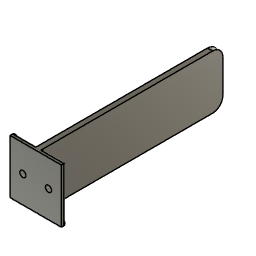
ear_bracket v2 (Autodesk Fusion 360 design; units mm, degrees)
Autodesk Fusion 360 part; units mm, degrees
sketch "Sketch1" plane through (0, 0, 0) normal (0, 1, 0) x (1, 0, 0)
  line L0 (10, -15) -> (-10, -15)
  line L1 (-10, -15) -> (-10, 6)
  line L2 (-10, 6) -> (10, 6)
  line L3 (10, 6) -> (10, -15)
  dimension "d1" = 21
  dimension "d2" = 20
  constraint horizontal L0
  constraint vertical L1
  constraint horizontal L2
  constraint vertical L3
  measures "d1" distance of L0.start L2.end
  measures "d2" distance of L0.start L0.end
extrude "Extrude1" add sketch "Sketch1" along normal blind 2
sketch "Sketch2" plane through (0, 2, 0) normal (0, 1, 0) x (-1, 0, 0)
  line L0 (-10, -6) -> (10, -6)
  line L1 (10, -6) -> (10, 15)
  line L2 (10, 15) -> (-10, 15)
  line L3 (-10, 15) -> (-10, -6)
  line L4 (-1, 15) -> (1, 15)
  line L5 (1, 15) -> (1, -6)
  line L6 (1, -6) -> (-1, -6)
  line L7 (-1, -6) -> (-1, 15)
  dimension "d5" = 2
  dimension "d6" = 9
  constraint horizontal L4
  constraint vertical L5
  constraint horizontal L6
  constraint vertical L7
  constraint coincident L0 L5.end
  constraint coincident L2 L4.start
  measures "d5" distance of L4.start L4.end
  measures "d6" distance of L1 L5
extrude "Extrude2" add sketch "Sketch2" along normal blind 70 contours L0 L2 L4 L5 L6 L7
sketch "Sketch3" plane through (0, 2, 0) normal (0, 1, 0) x (-1, 0, 0)
  line L0 (-1, -6) -> (-1, 15)
  line L1 (-1, 15) -> (-10, 15)
  line L2 (-10, 15) -> (-10, -6)
  line L3 (-10, -6) -> (-1, -6)
  circle A0 centre (-5, 4.5) radius 1.2
  circle A1 centre (5, 4.5) radius 1.2
  line L4 (10, 15) -> (1, 15)
  dimension "d9" = 2.4
  dimension "d10" = 2.4
  dimension "d11" = 10.5
  dimension "d12" = 10.5
  dimension "d19" = 10
  measures "d9" diameter of A0
  measures "d10" diameter of A1
  measures "d11" distance of A1.centre L4
  measures "d12" distance of L1 A0.centre
  measures "d19" distance of A0.centre A1.centre
extrude "Extrude3" cut sketch "Sketch3" against normal blind 2 contours A0 | A1
fillet "Fillet1" radius 1 6 edges at (10, 2, 4.5) (5.5, 2, 15) (-5.5, 2, 15) (-10, 2, 4.5) (-5.5, 2, -6) (5.5, 2, -6)
fillet "Fillet2" radius 4 2 edges at (0, 72, 15) (0, 72, -6)
